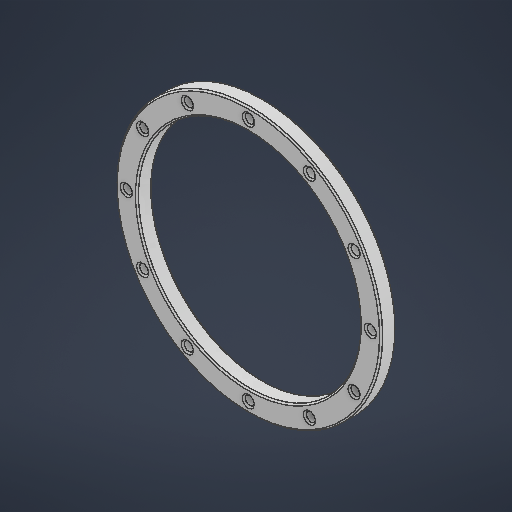
# Autodesk Inventor part: Фланец колеса
Saved by Autodesk Inventor 2025 (Build 290162010, 162A)
## iProperties
Created: 2025-01-17
Part Number: Фланец колеса
Material: Типовые
Document SubType Name: Modeling
Designer: Edward_Higgins
Density: 1 g/cm^3
Appearance: По умолчанию
Author: Edward_Higgins
Autodesk Inventor part; units mm, degrees
ref_plane "YZ Plane" through (0, 0, 0) normal (1, 0, 0) x (0, 1, 0)
ref_plane "XZ Plane" through (0, 0, 0) normal (0, 1, 0) x (-1, 0, 0)
ref_plane "XY Plane" through (0, 0, 0) normal (0, 0, 1) x (1, 0, 0)
sketch "Эскиз1" plane through (0, 0, 0) normal (0, 0, 1) x (1, 0, 0)
  circle A0 centre (0, 0) radius 43.5
  circle A1 centre (0, 0) radius 36.5
  dimension "d1" = 73
  dimension "d2" = 87
  constraints: 2 centre point, 2 coincident
  measures "d1" diameter of A1
  measures "d2" diameter of A0
extrude "Выдавливание1" add sketch "Эскиз1" along normal blind 5
sketch "Эскиз2" plane through (0, 0, 5) normal (0, 0, 1) x (1, 0, 0)
  circle A0 centre (0, 40) radius 1.5
  point P0 (0, 0)
  dimension "d5" = 40
  dimension "d6" = 3
  constraints: 1 centre point, 1 vertical alignment
  measures "d5" distance of point (0, 0) A0.centre
  measures "d6" diameter of A0
extrude "Выдавливание2" cut sketch "Эскиз2" against normal up to surface (5 mm away)
chamfer "Фаска2" distance 0.5 angle 45 2 edges at (-1.5, 40, 5) (-1.5, 40, 0)
pattern_circular "Круговой массив1" count 12 over 360 about axis through (0, 0, 0) along (0, 0, 1) of "Выдавливание2", "Фаска2"
chamfer "Фаска1" distance 0.5 angle 45 4 edges at (-43.5, 0, 5) (-43.5, 0, 0) (-36.5, 0, 5) (-36.5, 0, 0)
